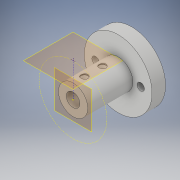
# Autodesk Inventor part: spannring_achse
Saved by Autodesk Inventor 2017 (Build 210142000, 142)
## iProperties
Part Number: spannring_achse
Material: Generisch
Document SubType Name: Modeling
Designer: Fabio
Density: 1 g/cm^3
Appearance: Vorgabe
Author: Fabio
Autodesk Inventor part; units mm, degrees
ref_plane "YZ Plane" through (0, 0, 0) normal (1, 0, 0) x (0, 1, 0)
ref_plane "XZ Plane" through (0, 0, 0) normal (0, 1, 0) x (-1, 0, 0)
ref_plane "XY Plane" through (0, 0, 0) normal (0, 0, 1) x (1, 0, 0)
sketch "Skizze1" plane through (0, 0, 0) normal (0, 1, 0) x (-1, 0, 0)
  circle A0 centre (0, 0) radius 15
  dimension "d0" = 30
  constraints: 1 centre point, 1 coincident
  measures "d0" diameter of A0
extrude "Extrusion1" add sketch "Skizze1" along normal blind 26
ref_plane "Arbeitsebene1" through (0, 26, 0) normal (0, 1, 0) x (1, 0, 0)
sketch "Skizze2" plane through (0, 26, 0) normal (0, 1, 0) x (1, 0, 0)
  circle A0 centre (0, 0) radius 15 projected
  circle A1 centre (0, 0) radius 15 construction
  circle A2 centre (0, 0) radius 15 construction
  line L0 (-10, 0) -> (10, 0) construction
  dimension "d42" = 10
  dimension "d43" = 10
  dimension "d44" = 20
  constraints: 2 coincident, 2 end point, 1 horizontal
  measures "d42" distance of point (0, 0) L0.start
  measures "d43" distance of point (0, 0) point (10, 0)
  measures "d44" distance of L0.end L0.start
ref_plane "Arbeitsebene2" through (0, 0, 0) normal (0, -1, 0) x (1, 0, 0)
sketch "Skizze3" plane through (0, 0, 0) normal (0, -1, 0) x (1, 0, 0)
  circle A0 centre (0, 0) radius 15 projected
  constraints: 1 coincident
hole "Bohrung2" at (0, 0, 0) direction (0, 1, 0) diameter 6 end through all
sketch "Skizze4" plane through (0, 0, 0) normal (0, -1, 0) x (1, 0, 0)
  point P0 (0, 0)
sketch "Skizze5" plane through (0, 0, 0) normal (0, -1, 0) x (1, 0, 0)
  line L0 (0, 0) -> (0, 15) construction
  circle A0 centre (0, 0) radius 15 construction
  constraints: 2 end point, 1 coincident, 1 vertical, 1 vertical alignment, 1 other
ref_plane "Arbeitsebene3" through (0, 0, 15) normal (0, 0, 1) x (1, 0, 0)
sketch "Skizze6" plane through (0, 0, 15) normal (0, 0, 1) x (1, 0, 0)
  line L0 (0, 0) -> (0, 27.6738) construction
  point P0 (0, 5)
  point P1 (0, 13)
  dimension "d25" = 8
  dimension "d26" = 5
  constraints: 2 end point, 2 point on line, 1 vertical
  measures "d25" distance of point (0, 13) point (0, 5)
  measures "d26" distance of L0.start point (0, 5)
hole "Bohrung3" at (0, 13, 15) at (0, 5, 15) direction (0, 0, -1) diameter 3 depth 9 tip angle 118
thread "Gewinde3" size "M3x0.5" class "6H" standard "ANSI Metric M Profile" full length
thread "Gewinde4" size "M3x0.5" class "6H" standard "ANSI Metric M Profile" full length
sketch "Skizze7" plane through (0, 0, 0) normal (0, -1, 0) x (1, 0, 0)
  circle A0 centre (0, 0) radius 6.5
  circle A1 centre (0, 0) radius 20
  dimension "d38" = 13
  dimension "d39" = 40
  constraints: 2 centre point, 2 coincident
  measures "d38" diameter of A0
  measures "d39" diameter of A1
extrude "Extrusion2" cut sketch "Skizze7" against normal blind 20
hole "Bohrung4" at (-10, 26, 0) at (10, 26, 0) direction (0, -1, 0) diameter 3.3 end through all
